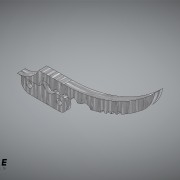
# Autodesk Inventor part: シールド殺し
Saved by Autodesk Inventor 2020 (Build 240168000, 168)
## iProperties
Created: 2019-12-03
Part Number: シールド殺し
Material: アルミニウム 7075
Document SubType Name: Modeling
Designer: tanjihayato
Density: 2.81 g/cm^3
Appearance: サテン - ブラシ仕上げ 重厚
Mass: 4.13611 g
Surface Area: 16.6487 cm^2
Volume: 1.47192 cm^3
Author: tanjihayato
Autodesk Inventor part; units mm, degrees
ref_plane "YZ Plane" through (0, 0, 0) normal (1, 0, 0) x (0, 1, 0)
ref_plane "XZ Plane" through (0, 0, 0) normal (0, 1, 0) x (-1, 0, 0)
ref_plane "XY Plane" through (0, 0, 0) normal (0, 0, 1) x (1, 0, 0)
sketch "スケッチ1" plane through (0, 0, 0) normal (0, 0, 1) x (1, 0, 0)
  circle A0 centre (0, 0) radius 2
  circle A1 centre (15, 0) radius 2
  arc A2 (-0.2273, 4.9948) -> (-3.6359, -3.4322) centre (0, 0) ccw
  circle A3 centre (55, 0) radius 2
  circle A4 centre (43.6863, -14) radius 2
  circle A5 centre (55, 0) radius 5.025
  arc A6 (58.5132, 7.2151) -> (53.7727, 7.9306) centre (55, 0) ccw
  arc A7 (47.9053, -14.5126) -> (46.3576, -10.6944) centre (43.6863, -14) ccw
  line L0 (80, -19) -> (95, -19)
  circle A8 centre (95, -15) radius 2
  circle A9 centre (80, -15) radius 2
  arc A10 (95, -19) -> (96.7511, -11.4037) centre (95, -15) ccw
  circle A11 centre (80, -15) radius 4 construction
  line L1 (55.7328, -19) -> (80, -19)
  line L2 (58.5132, 7.2151) -> (96.7511, -11.4037)
  arc A12 (41.3268, -1.451) -> (46.3576, -10.6944) centre (55, 0) ccw
  arc A13 (60.1221, -5.4785) -> (54.6591, 7.4922) centre (55, 0) ccw
  line L3 (-0.2273, 4.9948) -> (54.6591, 7.4922)
  circle A14 centre (13, -14.5) radius 1.5
  arc A15 (9.7277, -17.589) -> (13, -19) centre (13, -14.5) ccw
  line L4 (-3.6359, -3.4322) -> (9.7277, -17.589)
  arc A16 (43.6863, -19) -> (47.101, -17.6524) centre (43.6863, -14) ccw
  line L5 (47.9053, -14.5126) -> (53.1517, -18.1862)
  line L6 (13, -19) -> (43.6863, -19)
  line L7 (47.101, -17.6524) -> (60.1221, -5.4785)
  circle A17 centre (66.8562, -1.8523) radius 1.5
  circle A18 centre (66.8562, -1.8523) radius 4.5 construction
  arc A19 (41.3268, -1.451) -> (37.1005, 2.3505) centre (37.1005, -1.8995) ccw
  line L8 (37.1005, 5.3505) -> (53.7727, 7.9306)
  line L9 (37.1005, 5.3505) -> (37.1005, 2.3505)
  circle A20 centre (55.7328, -14.5) radius 1.5
  arc A21 (53.1517, -18.1862) -> (55.7328, -19) centre (55.7328, -14.5) ccw
  arc A22 (80, -11) -> (80, -19) centre (80, -15) ccw
  line L10 (358.0202, -11) -> (380, -19)
  line L11 (380, -19) -> (80, -19)
  circle A23 centre (348.0202, -15) radius 1.25
  circle A24 centre (333.0202, -15) radius 1.25
  circle A25 centre (318.0202, -15) radius 1.25
  circle A26 centre (303.0202, -15) radius 1.25
  line L12 (80, -11) -> (207.8755, -11)
  line L13 (358.0202, -11) -> (248.9511, -11)
  arc A27 (213.7823, -10) -> (213.8378, -11) centre (210.8567, -10.6639) ccw
  line L14 (213.7823, -10) -> (214.7761, -9.8894)
  line L15 (213.8378, -11) -> (214.8378, -11)
  line L16 (219.357, -11) -> (218.357, -11)
  line L17 (218.2737, -9.5) -> (219.2676, -9.3894)
  line L18 (222.8762, -11) -> (223.8762, -11)
  line L19 (222.7652, -9) -> (223.7591, -8.8894)
  arc A28 (214.8378, -11) -> (218.357, -11) centre (216.5974, -10.3453) ccw
  arc A29 (218.2737, -9.5) -> (214.7761, -9.8894) centre (216.5974, -10.3453) ccw
  arc A30 (219.357, -11) -> (222.8762, -11) centre (221.1166, -10.0946) ccw
  arc A31 (222.7652, -9) -> (219.2676, -9.3894) centre (221.1166, -10.0946) ccw
  line L20 (210.8567, -10.6639) -> (233.0155, -9.4343) construction
  arc A32 (223.8762, -11) -> (229.892, -10.6107) centre (226.7628, -8.9308) ccw
  arc A33 (226.8407, -8.7739) -> (223.7591, -8.8894) centre (225.3075, -9.0352) ccw
  arc A34 (226.8407, -8.7739) -> (230.4998, -7.0068) centre (226.5478, -3.4953) ccw
  arc A35 (233.6316, -8.397) -> (230.4998, -7.0068) centre (231.2455, -9.5496) ccw
  arc A36 (235.4619, -12.6053) -> (229.892, -10.6107) centre (230.3136, -18.2076) ccw
  arc A37 (235.4619, -12.6053) -> (239.6511, -11) centre (234.0497, -2.6513) ccw
  arc A38 (259.6965, 4.4867) -> (265.8152, 14.9495) centre (248.2498, 18.2013) ccw
  arc A39 (220.191, -4.195) -> (265.8152, 14.9495) centre (219.3797, 61.6752) ccw
  line L21 (220.191, -4.195) -> (207.615, -4.3499)
  arc A40 (196.7777, -11) -> (207.615, -4.3499) centre (196.7777, 1.1554) ccw
  line L22 (222.8762, -11) -> (240.076, -10.0456) construction
  line L23 (222.7652, -9) -> (239.478, -8.0726) construction
  line L24 (239.6511, -11) -> (240.6511, -11)
  arc A41 (240.6511, -11) -> (242.7511, -11) centre (241.7011, -11) ccw
  line L25 (242.7511, -11) -> (243.7511, -11)
  arc A42 (243.7511, -11) -> (245.8511, -11) centre (244.8011, -11) ccw
  line L26 (245.8511, -11) -> (246.8511, -11)
  arc A43 (246.8511, -11) -> (248.9511, -11) centre (247.9011, -11) ccw
  arc A44 (240.735, -6.337) -> (238.7449, -7.0075) centre (239.7428, -6.6807) ccw
  arc A45 (243.5362, -5.2633) -> (241.5809, -6.0291) centre (242.5618, -5.6544) ccw
  arc A46 (246.2823, -4.0554) -> (244.3663, -4.9148) centre (245.3279, -4.4932) ccw
  arc A47 (248.9668, -2.7162) -> (247.0946, -3.6672) centre (248.0347, -3.1996) ccw
  arc A48 (233.6316, -8.397) -> (238.7449, -7.0075) centre (219.9279, 52.1342) ccw
  arc A49 (240.735, -6.337) -> (241.5809, -6.0291) centre (219.9279, 52.1342) ccw
  arc A50 (243.5362, -5.2633) -> (244.3663, -4.9148) centre (219.9279, 52.1342) ccw
  arc A51 (246.2823, -4.0554) -> (247.0946, -3.6672) centre (219.9279, 52.1342) ccw
  arc A52 (248.9668, -2.7162) -> (259.6965, 4.4867) centre (219.9279, 52.1342) ccw
  line L27 (196.7777, -11) -> (196.7777, -15)
  circle A53 centre (200.7777, -15) radius 1.25
  circle A54 centre (215.7777, -15) radius 1.25
  arc A55 (196.7777, -15) -> (200.7777, -19) centre (200.7777, -15) ccw
  arc A56 (215.7777, -19) -> (217.9536, -11.6436) centre (215.7777, -15) ccw
  circle A57 centre (200.7777, -15) radius 1.5
  circle A58 centre (215.7777, -15) radius 1.5
  line L28 (200.7777, -19) -> (215.7777, -19)
  dimension "d0" = 4
  dimension "d1" = 4
  dimension "d2" = 15
  dimension "d3" = 3
  dimension "d4" = 4
  dimension "d5" = 4
  dimension "d6" = 10.05
  dimension "d7" = 3
  dimension "d8" = 8.5
  dimension "d9" = 4
  dimension "d10" = 4
  dimension "d11" = 15
  dimension "d12" = 15
  dimension "d13" = 3
  dimension "d14" = 3
  dimension "d15" = 3
  dimension "d16" = 35
  dimension "d17" = 3
  dimension "d18" = 40
  dimension "d19" = 40
  dimension "d20" = 18
  dimension "d21" = 15
  dimension "d22" = 13
  dimension "d23" = 8.5
  dimension "d24" = 18
  dimension "d25" = 45
  dimension "d26" = 3
  dimension "d27" = 3
  dimension "d28" = 3
  dimension "d29" = 3
  dimension "d30" = 8
  dimension "d31" = 380
  dimension "d32" = 20
  dimension "d33" = 4
  dimension "d34" = 8
  dimension "d35" = 2.5
  dimension "d36" = 2.5
  dimension "d37" = 2.5
  dimension "d38" = 2.5
  dimension "d39" = 4
  dimension "d40" = 15
  dimension "d41" = 15
  dimension "d42" = 15
  dimension "d43" = 10
  dimension "d44" = 6
  dimension "d45" = 1
  dimension "d46" = 1.5
  dimension "d47" = 1
  dimension "d48" = 1
  dimension "d49" = 1
  dimension "d50" = 2
  dimension "d51" = 1
  dimension "d52" = 1.0015
  dimension "d53" = 1.0015
  dimension "d54" = 0.7511
  dimension "d55" = 0.7511
  dimension "d56" = 3.176
  dimension "d57" = 3.176
  dimension "d58" = 1.05
  dimension "d59" = 1.05
  dimension "d60" = 1.05
  dimension "d61" = 1
  dimension "d62" = 1
  dimension "d63" = 1
  constraints: 91 point on circle, 59 centre point, 58 end point, 30 tangent, 13 point on line, 12 coincident, 9 horizontal, 8 collinear, 6 horizontal alignment, 2 concentric, 2 vertical, 1 parallel, 2 other
  measures "d0" diameter of A0
  measures "d1" diameter of A1
  measures "d2" distance of point (0, 0) A1.centre
  measures "d3" radial gap between concentric circles of A0 A2
  measures "d4" diameter of A3
  measures "d5" diameter of A4
  measures "d6" diameter of A5
  measures "d7" radial gap between concentric circles of A5 A6
  measures "d8" diameter of A7
  measures "d9" diameter of A8
  measures "d10" diameter of A9
  measures "d11" distance of A9.centre A8.centre
  measures "d12" diameter of A13
  measures "d13" diameter of A14
  measures "d14" radial gap between concentric circles of A14 A15
  measures "d15" radial gap between concentric circles of A16 A4
  measures "d16" angle of L1 L5
  measures "d17" diameter of A17
  measures "d18" distance of A5.centre A1.centre
  measures "d19" horizontal distance of A3.centre A8.centre
  measures "d20" distance of A3.centre A4.centre
  measures "d21" vertical distance of A9.centre A3.centre
  measures "d22" horizontal distance of A14.centre point (0, 0)
  measures "d23" diameter of A19
  measures "d24" distance of A19.centre A3.centre
  measures "d26" distance of L8.start L9.end
  measures "d27" diameter of A20
  measures "d28" radial gap between concentric circles of A18 A17
  measures "d29" radial gap between concentric circles of A20 A21
  measures "d30" diameter of A22
  measures "d31" horizontal distance of point (0, 0) L10.end
  measures "d32" angle of L11 L10
  measures "d33" radius of A10
  measures "d34" diameter of A11
  measures "d35" diameter of A23
  measures "d36" diameter of A24
  measures "d37" diameter of A25
  measures "d38" diameter of A26
  measures "d39" distance from line of L11 A26.centre
  measures "d40" distance of A25.centre A26.centre
  measures "d41" distance of A25.centre A24.centre
  measures "d42" distance of A23.centre A24.centre
  measures "d43" horizontal distance of A23.centre L10.start
  measures "d44" diameter of A27
  measures "d45" vertical distance of L15.start L14.start
  measures "d46" vertical distance of L16.end L17.start
  measures "d47" distance of L15.start L15.end
  measures "d48" distance of L16.end L16.start
  measures "d49" distance of L18.start L18.end
  measures "d50" vertical distance of L18.start L19.start
  measures "d51" distance of L19.start L19.end
  measures "d52" distance from line of L20 L19.start
  measures "d53" distance from line of L18.start L20
  measures "d54" distance from line of L20 L17.start
  measures "d55" distance from line of L20 L16.end
  measures "d56" angle of L19 L23
  measures "d57" angle of L18 L22
  measures "d58" radius of A41
  measures "d59" radius of A42
  measures "d60" radius of A43
  measures "d61" distance of L26.start L26.end
  measures "d62" distance of L25.start L25.end
  measures "d63" distance of L24.start L24.end
extrude "押し出し1" add sketch "スケッチ1" along normal blind 4 contours A40 L21 A39 A38 A52 A47 A51 A46 A50 A45 A49 A44 A48 A35 A34 A33 L19 A31 L17 A29 L14 A27 L12
extrude "押し出し2" add sketch "スケッチ1" along normal blind 2 contours L12 A27 L15 A28 A56 L11 A55 L27
sketch "スケッチ2" plane through (0, 0, 0) normal (0, 0, -1) x (-1, 0, 0)
  circle A0 centre (-200.7777, -15) radius 1.5 projected
  circle A1 centre (-215.7777, -15) radius 1.5 projected
  arc A2 (-213.8378, -11) -> (-213.7823, -10) centre (-210.8567, -10.6639) ccw projected
  line L0 (-214.8378, -11) -> (-213.8378, -11) projected
  arc A3 (-217.9536, -11.6436) -> (-214.8378, -11) centre (-216.5974, -10.3453) ccw projected
  arc A4 (-217.9536, -11.6436) -> (-215.7777, -19) centre (-215.7777, -15) ccw projected
  line L1 (-200.7777, -19) -> (-215.7777, -19) projected
  arc A5 (-200.7777, -19) -> (-196.7777, -15) centre (-200.7777, -15) ccw projected
  line L2 (-196.7777, -11) -> (-196.7777, -15) projected
  arc A6 (-207.615, -4.3499) -> (-196.7777, -11) centre (-196.7777, 1.1554) ccw projected
  line L3 (-220.191, -4.195) -> (-207.615, -4.3499) projected
  arc A7 (-265.8152, 14.9495) -> (-220.191, -4.195) centre (-219.3797, 61.6752) ccw projected
  arc A8 (-265.8152, 14.9495) -> (-259.6965, 4.4867) centre (-248.2498, 18.2013) ccw projected
  arc A9 (-259.6965, 4.4867) -> (-248.9668, -2.7162) centre (-219.9279, 52.1342) ccw projected
  arc A10 (-247.0946, -3.6672) -> (-248.9668, -2.7162) centre (-248.0347, -3.1996) ccw projected
  arc A11 (-247.0946, -3.6672) -> (-246.2823, -4.0554) centre (-219.9279, 52.1342) ccw projected
  arc A12 (-244.3663, -4.9148) -> (-246.2823, -4.0554) centre (-245.3279, -4.4932) ccw projected
  arc A13 (-244.3663, -4.9148) -> (-243.5362, -5.2633) centre (-219.9279, 52.1342) ccw projected
  arc A14 (-241.5809, -6.0291) -> (-243.5362, -5.2633) centre (-242.5618, -5.6544) ccw projected
  arc A15 (-241.5809, -6.0291) -> (-240.735, -6.337) centre (-219.9279, 52.1342) ccw projected
  arc A16 (-238.7449, -7.0075) -> (-240.735, -6.337) centre (-239.7428, -6.6807) ccw projected
  arc A17 (-238.7449, -7.0075) -> (-233.6316, -8.397) centre (-219.9279, 52.1342) ccw projected
  arc A18 (-230.4998, -7.0068) -> (-233.6316, -8.397) centre (-231.2455, -9.5496) ccw projected
  arc A19 (-230.4998, -7.0068) -> (-226.8407, -8.7739) centre (-226.5478, -3.4953) ccw projected
  arc A20 (-223.7591, -8.8894) -> (-226.8407, -8.7739) centre (-225.3075, -9.0352) ccw projected
  line L4 (-222.7652, -9) -> (-223.7591, -8.8894) projected
  arc A21 (-219.2676, -9.3894) -> (-222.7652, -9) centre (-221.1166, -10.0946) ccw projected
  line L5 (-218.2737, -9.5) -> (-219.2676, -9.3894) projected
  arc A22 (-214.7761, -9.8894) -> (-218.2737, -9.5) centre (-216.5974, -10.3453) ccw projected
  line L6 (-213.7823, -10) -> (-214.7761, -9.8894) projected
  arc A23 (-213.8378, -11) -> (-207.8755, -11) centre (-210.8567, -10.6639) ccw projected
  circle A24 centre (-214.2944, -10.9995) radius 1.05
  arc A25 (-217.9536, -11.6436) -> (-214.8378, -11) centre (-216.5974, -10.3453) ccw projected
  arc A26 (-212.9299, -12.8322) -> (-216.0149, -12.1301) centre (-215.059, -15.0588) ccw
  arc A27 (-217.9536, -11.6436) -> (-214.8378, -11) centre (-216.5974, -10.3453) ccw projected
  point P0 (0, 0)
  point P1 (-216.0149, -12.1301)
  point P2 (-212.9299, -12.8322)
  dimension "d83" = 2.1
  constraints: 4 point on circle, 4 tangent, 2 centre point, 1 other
  measures "d83" diameter of A24
extrude "押し出し3" cut sketch "スケッチ2" against normal blind 10 contours A26 A24 A2 | A24 A3 L0 A2 | A26 A3 A24 picked at (-214.4032, -11.5037)
fillet "フィレット1" radius 1 1 edges at (217.9536, -11.6436, 1)
equation "\"d53\" = d52"
equation "\"d55\" = d54"
equation "\"d57\" = d56"
